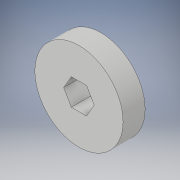
# Autodesk Inventor part: RobotArm Washer
Saved by Autodesk Inventor 2018 (Build 220112000, 112)
## iProperties
Created: 2018-01-13
Part Number: RobotArm Washer
Material: Generic
Document SubType Name: Modeling
Designer: lopez.xavier
Density: 1 g/cm^3
Appearance: Default
Author: lopez.xavier
Autodesk Inventor part; units mm, degrees
ref_plane "YZ Plane" through (0, 0, 0) normal (1, 0, 0) x (0, 1, 0)
ref_plane "XZ Plane" through (0, 0, 0) normal (0, 1, 0) x (-1, 0, 0)
ref_plane "XY Plane" through (0, 0, 0) normal (0, 0, 1) x (1, 0, 0)
sketch "Sketch1" plane through (0, 0, 0) normal (0, 0, 1) x (1, 0, 0)
  circle A0 centre (0, 0) radius 12.7
  line L0 (2.1997, 3.81) -> (4.3994, 0)
  line L1 (4.3994, 0) -> (2.1997, -3.81)
  line L2 (2.1997, -3.81) -> (-2.1997, -3.81)
  line L3 (-2.1997, -3.81) -> (-4.3994, 0)
  line L4 (-4.3994, 0) -> (-2.1997, 3.81)
  line L5 (-2.1997, 3.81) -> (2.1997, 3.81)
  line L6 (0, 0) -> (1.0545, 0)
  dimension "d0" = 25.4
  dimension "d1" = 7.62
  constraints: 14 end point, 2 coincident, 1 centre point, 1 horizontal, 1 parallel, 13 other
  measures "d0" diameter of A0
  measures "d1" distance between parallel lines of L2 L5
extrude "Extrusion1" add sketch "Sketch1" along normal blind 6.35
body "Solid1"
